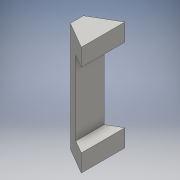
# Autodesk Inventor part: cable_tie_bracket
Saved by Autodesk Inventor 2016 (Build 200138000, 138)
## iProperties
Created: 2016-05-19
Part Number: cable_tie_bracket
Material: Generic
Document SubType Name: Modeling
Designer: MAS Staff
Density: 1 g/cm^3
Appearance: Default
Author: MAS Staff
Autodesk Inventor part; units mm, degrees
ref_plane "YZ Plane" through (0, 0, 0) normal (1, 0, 0) x (0, 1, 0)
ref_plane "XZ Plane" through (0, 0, 0) normal (0, 1, 0) x (-1, 0, 0)
ref_plane "XY Plane" through (0, 0, 0) normal (0, 0, 1) x (1, 0, 0)
sketch "Sketch1" plane through (0, 0, 0) normal (0, 1, 0) x (-1, 0, 0)
  line L0 (0, 0) -> (6, 0)
  line L1 (6, 0) -> (6, -25)
  line L2 (6, -25) -> (0, -25)
  line L3 (0, -25) -> (0, 0)
  line L4 (0, -21) -> (0, -4)
  dimension "d0" = 25
  dimension "d1" = 6
  constraints: 10 end point, 2 parallel, 1 horizontal, 1 perpendicular, 1 point on line
  measures "d0" distance between parallel lines of L0 L2
  measures "d1" distance between parallel lines of L3 L1
sketch "Sketch2" plane through (0, 0, 0) normal (0, 0, 1) x (1, 0, 0)
  line L0 (0, 0) -> (-6, 0)
  line L1 (-6, 0) -> (-6, 10)
  line L2 (-6, 10) -> (0, 10)
  line L3 (0, 10) -> (0, 0)
  line L4 (0, 0) -> (-6, 3.5)
  line L5 (0, 10) -> (-6, 6.5)
  dimension "d5" = 10
  dimension "d6" = 6
  dimension "d13" = 3.5
  dimension "d14" = 3.5
  constraints: 12 end point, 2 parallel, 2 point on line, 1 horizontal, 1 perpendicular
  measures "d5" distance between parallel lines of L0 L2
  measures "d6" distance between parallel lines of L1 L3
  measures "d13" distance from line of L0 L4.end
  measures "d14" distance of L1.end L5.end
sketch "Sketch3" plane through (0, 0, 0) normal (0, 1, 0) x (-1, 0, 0)
  line L0 (0, -4) -> (3, -4)
  line L1 (3, -4) -> (3, -21)
  line L2 (3, -21) -> (0, -21)
  line L3 (0, -21) -> (0, -4)
  point P0 (0, 0)
  dimension "d7" = 4
  dimension "d8" = 3
  dimension "d9" = 21
  dimension "d10" = 0
  constraints: 8 end point, 2 parallel, 1 horizontal, 1 perpendicular
  measures "d7" distance from line of point (0, 0) L0
  measures "d8" distance between parallel lines of L3 L1
  measures "d9" distance from line of point (0, 0) L2
  measures "d10" distance from line of point (0, 0) L3
extrude "Extrusion1" add sketch "Sketch1" along normal blind 10
extrude "Extrusion2" cut sketch "Sketch3" along normal blind 10
extrude "Extrusion3" cut sketch "Sketch2" against normal blind 25 contours L5 L1 L2
extrude "Extrusion4" cut sketch "Sketch2" against normal blind 25 contours L0 L1 L4
equation "\"d6\" = d1"
equation "\"d13\" = d14"
equation "\"d9\" = d0 - d7"
equation "\"d11\" = d5"
equation "\"d15\" = d5"
equation "\"d17\" = d0"
equation "\"d19\" = d0"
body "Solid1"
